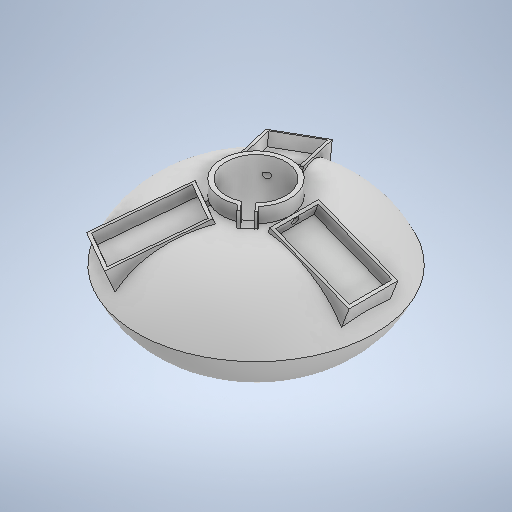
# Autodesk Inventor part: Water Sensor Bouy
Saved by Autodesk Inventor 2025 (Build 290162000, 162)
## iProperties
Created: 2024-06-17
Part Number: Water Sensor Bouy
Material: Generic
Document SubType Name: Modeling
Designer: track
Density: 1 g/cm^3
Appearance: Default
Author: track
## iProperties of the stored document Water Sensor Bouy_3DPrint.ipt
Created: 2024-06-17
Part Number: Water Sensor Bouy_3DPrint
Material: Generic
Document SubType Name: Modeling
Designer: track
Density: 1 g/cm^3
Appearance: Default
Author: track
Autodesk Inventor part; units mm, degrees
ref_plane "YZ Plane" through (0, 0, 0) normal (1, 0, 0) x (0, 1, 0)
ref_plane "XZ Plane" through (0, 0, 0) normal (0, 1, 0) x (-1, 0, 0)
ref_plane "XY Plane" through (0, 0, 0) normal (0, 0, 1) x (1, 0, 0)
sketch "Sketch1" plane through (0, 0, 0) normal (0, 0, 1) x (1, 0, 0)
  line L0 (0, 0) -> (0, 76.2)
  line L1 (25.3, 0) -> (25.3, 101.6)
  line L2 (25.3, 50.8) -> (101.5, 50.8)
  arc A0 (101.5, 50.8) -> (25.3, 101.6) centre (25.3, 19.05) ccw
  arc A1 (25.3, 0) -> (101.5, 50.8) centre (25.3, 82.55) ccw
  line L3 (35.3, 90.9075) -> (35.3, 10.6925)
  arc A2 (35.3, 10.6925) -> (90.5337, 50.8) centre (25.3, 82.55) ccw
  arc A3 (90.5337, 50.8) -> (35.3, 90.9075) centre (25.3, 19.05) ccw
  point P0 (25.3, 25.4)
  point P1 (84.8683, 25.4)
  point P2 (35.3, 31.75)
  point P3 (77.0964, 31.75)
  point P4 (35.3, 50.8)
  point P5 (90.5337, 50.8)
  point P6 (90.5337, 50.8)
  dimension "d0" = 101.6
  dimension "d1" = 25.3
  dimension "d2" = 50.8
  dimension "d3" = 0
  dimension "d4" = 76.2
  dimension "d24" = 82.55
  dimension "d33" = 10
  constraints: 10 point on circle, 8 end point, 4 centre point, 4 point on line, 2 vertical, 1 horizontal, 1 midpoint, 2 other
  measures "d0" distance of L1.start L1.end
  measures "d1" distance between parallel lines of L1 L0
  measures "d2" distance from line of L1.end L2
  measures "d3" vertical distance of L0.start L1.start
  measures "d4" distance of L2.start L2.end
  measures "d24" radius of A0
  measures "d33" distance between parallel lines of L1 L3
revolve "Revolution1" add sketch "Sketch1" angle 360 about axis through (0, 0, 0) along (0, 1, 0) contours L1 L2 L3 A2 A1 | L1 A0 L2 A3 L3
sketch "Sketch6" plane through (0, 0, 0) normal (0, 0, 1) x (1, 0, 0)
  arc A0 (101.5, 50.8) -> (25.3, 101.6) centre (25.3, 19.05) ccw projected
  line L0 (25.3, 101.6) -> (-25.3, 101.6) projected
  arc A1 (96.42, 60.96) -> (25.3, 101.6) centre (25.3, 19.05) ccw
  line L1 (55.0851, 96.0393) -> (28.9662, 50.8)
  line L2 (90.5337, 50.8) -> (-90.5337, 50.8) projected
  point P0 (0, 0)
  dimension "d34" = 60
  dimension "d35" = 12.7
  constraints: 4 point on circle, 2 end point, 1 centre point, 1 concentric, 1 point on line
  measures "d34" angle of L2 L1
  measures "d35" distance from line of A0.centre L1
ref_plane "Work Plane4" through (55.0851, 96.0393, 0) normal (0.3608127, 0.9326383, 0) x (-0.9326383, 0.3608127, 0)
sketch "Sketch17" plane through (55.0851, 96.0393, 0) normal (0.3608127, 0.9326383, 0) x (-0.9326383, 0.3608127, 0)
  line L0 (21.6308, 18.25) -> (-45.8692, 18.25)
  line L1 (-45.8692, 18.25) -> (-45.8692, -18.25)
  line L2 (-45.8692, -18.25) -> (21.6308, -18.25)
  line L3 (21.6308, -18.25) -> (21.6308, 18.25)
  ellipse E0 centre (53.3808, 0) end of major axis (53.3808, -25.3) minor radius 23.5957 projected
  point P0 (16.7223, 0)
  point P1 (21.6308, 0)
  dimension "d93" = 36.5
  dimension "d94" = 67.5
  dimension "d95" = 0
  dimension "d96" = 31.75
  constraints: 8 end point, 2 parallel, 1 horizontal, 1 midpoint, 1 perpendicular
  measures "d93" distance of L2.end L0.start
  measures "d94" distance of L1.end L2.end
  measures "d95" vertical distance of E0.centre point (21.631, 0)
  measures "d96" distance from line of E0.centre L3
extrude "Extrusion10" cut sketch "Sketch17" against normal blind 10 contours L3 L2 L1 L0
sketch "Sketch18" plane through (55.0851, 96.0393, 0) normal (0.3608127, 0.9326383, 0) x (-0.9326383, 0.3608127, 0)
  line L0 (21.6308, -18.25) -> (-36.2714, -18.25) projected
  line L1 (21.6308, -18.25) -> (-45.8692, -18.25)
  line L2 (-45.8692, -18.25) -> (-45.8692, 18.25)
  line L3 (-45.8692, 18.25) -> (21.6308, 18.25)
  line L4 (21.6308, 18.25) -> (21.6308, -18.25)
  line L5 (24.1708, -20.79) -> (-48.4092, -20.79)
  line L6 (-48.4092, -20.79) -> (-48.4092, 20.79)
  line L7 (-48.4092, 20.79) -> (24.1708, 20.79)
  line L8 (24.1708, 20.79) -> (24.1708, -20.79)
  point P0 (16.7223, 0)
  dimension "d99" = 36.5
  dimension "d100" = 67.5
  dimension "d101" = 2.54
  constraints: 16 end point, 4 parallel, 2 perpendicular, 1 horizontal, 3 other
  measures "d99" distance of L3.end L0.start
  measures "d100" distance of L0.start L1.end
  measures "d101" distance between parallel lines of L3 L7
extrude "Extrusion11" add sketch "Sketch18" against normal up to surface
sketch "Sketch19" plane through (51.477, 86.7129, 0) normal (0.3608127, 0.9326383, 0) x (0.9326383, -0.3608127, 0)
  line L0 (45.8692, -18.25) -> (-21.6308, -18.25) projected
  line L1 (-21.6308, 18.25) -> (36.2714, 18.25) projected
  line L2 (45.8692, -18.25) -> (-21.6308, -18.25)
  line L3 (-21.6308, -18.25) -> (-21.6308, 18.25)
  line L4 (-21.6308, 18.25) -> (45.8692, 18.25)
  line L5 (45.8692, 18.25) -> (45.8692, -18.25)
  point P0 (-16.7223, 0)
  point P1 (-21.6308, -18.25)
  constraints: 8 end point, 2 parallel, 1 horizontal, 1 perpendicular
extrude "Extrusion12" add sketch "Sketch19" against normal blind 10
sketch "Sketch20" plane through (0, 0, 0) normal (1, 0, 0) x (0, 1, 0)
  circle A0 centre (100.034, 0) radius 3
  line L0 (101.6, -25.3) -> (101.6, 25.3) projected
  line L1 (103.844, 18.25) -> (103.844, -18.25) projected
  line L2 (103.844, -18.25) -> (94.5176, -18.25) projected
  point P0 (0, 0)
  dimension "d106" = 6
  dimension "d108" = 3.81
  dimension "d109" = 18.25
  constraints: 1 centre point
  measures "d106" diameter of A0
  measures "d108" distance from line of L1 A0.centre
  measures "d109" distance from line of L2 A0.centre
extrude "Extrusion13" cut sketch "Sketch20" against normal up to surface surface through (34.9113, 103.844, 18.25) normal (-0.9326383, 0.3608127, 0)
pattern_circular "Circular Pattern4" count 3 over 360 about axis through (0, 50.8, 0) along (0, 1, 0) of "Extrusion13", "Extrusion12", "Extrusion11", "Extrusion10"
sketch "Sketch21" plane through (0, 0, 0) normal (1, 0, 0) x (0, 1, 0)
  arc A0 (50.8, -101.5) -> (101.6, -25.3) centre (19.05, -25.3) ccw projected
  arc A1 (50.8, -101.5) -> (101.6, -25.3) centre (19.05, -25.3) ccw
  line L0 (101.6, -25.3) -> (114.3, -25.3)
  line L1 (114.3, -25.3) -> (114.3, -29.11)
  line L2 (114.3, -29.11) -> (101.512, -29.11)
  line L3 (0, 0) -> (101.6, 0)
  line L4 (101.6, -20.5187) -> (101.6, 20.5187) projected
  dimension "d115" = 3.81
  dimension "d116" = 12.7
  dimension "d117" = 25.3
  dimension "d118" = 25.3
  constraints: 8 end point, 5 point on circle, 2 perpendicular, 1 centre point, 1 horizontal, 1 midpoint
  measures "d115" distance of L0.end L1.end
  measures "d116" distance of L0.start L0.end
  measures "d117" distance between parallel lines of L3 L0
  measures "d118" distance from line of L3 A0.centre
revolve "Revolution3" add sketch "Sketch21" angle 210 about axis through (0, 0, 0) along (0, 1, 0) and the other way 140
sketch "Sketch22" plane through (18.7115, 114.3, 22.2996) normal (0, 1, 0) x (0.7660444, 0, -0.6427876)
  line L0 (0, 29.11) -> (-2.205, 3.9063)
  arc A0 (0, 3.81) -> (-4.3933, 4.1944) centre (0, 29.11) ccw projected
  line L1 (0, 29.11) -> (0, 54.41)
  circle A1 centre (0, 29.11) radius 25.3
  dimension "d121" = 175
  constraints: 4 end point, 1 coincident, 1 point on circle, 1 vertical, 3 other
  measures "d121" angle of L1 L0
ref_plane "Work Plane5" through (14.5115, 114.3, 20.7245) normal (-0.7660444, 0, 0.6427876) x (0.6427876, 0, 0.7660444)
sketch "Sketch23" plane through (14.5115, 114.3, 20.7245) normal (-0.7660444, 0, 0.6427876) x (0.6427876, 0, 0.7660444)
  line L0 (-0.2881, -12.7) -> (-0.2881, 0) projected
  line L1 (-0.2881, 0) -> (8.6019, 0)
  line L2 (8.6019, 0) -> (8.6019, -15.24)
  line L3 (8.6019, -15.24) -> (-0.2881, -15.24)
  line L4 (-0.2881, -15.24) -> (-0.2881, 0)
  point P0 (-25.2037, -114.3)
  point P1 (-0.2881, -12.7)
  dimension "d122" = 8.89
  dimension "d123" = 15.24
  constraints: 8 end point, 2 parallel, 1 horizontal, 1 perpendicular
  measures "d122" distance of L0.end L1.end
  measures "d123" distance of L1.end L2.end
extrude "Extrusion14" add sketch "Sketch23" along normal mid plane 12.7
sketch "Sketch24" plane through (15.1763, 101.0432, 31.3957) normal (0.6427876, 0, 0.7660444) x (0.7660444, 0, -0.6427876)
  line L0 (33.855, 13.2568) -> (-16.745, 13.2568) projected
  line L1 (1.905, 13.2568) -> (10.795, 13.2568)
  line L2 (10.795, 13.2568) -> (10.795, -0.2814)
  line L3 (10.795, -0.2814) -> (1.905, -0.2814)
  line L4 (1.905, -0.2814) -> (1.905, 13.2568)
  line L5 (12.7, 13.2568) -> (12.7, 0.0908) projected
  line L6 (0, 0) -> (0, 13.2568) projected
  point P0 (8.555, -101.0432)
  point P1 (4.1617, 13.2568)
  point P2 (10.795, 13.2568)
  dimension "d126" = 1.905
  dimension "d127" = 1.905
  dimension "d128" = 13.5382
  constraints: 8 end point, 2 parallel, 1 horizontal, 1 perpendicular, 1 point on line
  measures "d126" distance between parallel lines of L5 L2
  measures "d127" distance between parallel lines of L6 L4
  measures "d128" distance of L1.end L2.end
extrude "Extrusion15" cut sketch "Sketch24" against normal blind 12.7
sketch "Sketch25" plane through (19.3759, 114.3, 16.6428) normal (0.7660444, 0, -0.6427876) x (-0.6427876, 0, -0.7660444)
  circle A0 centre (-6.0619, -2.54) radius 0.75
  circle A1 centre (-6.0619, -5.08) radius 0.75
  circle A2 centre (-6.0619, -7.62) radius 0.75
  line L0 (-8.6019, 0) -> (-8.6019, -13.166) projected
  line L1 (-3.6097, 0) -> (-8.6019, 0) projected
  point P0 (25.2037, -114.3)
  dimension "d131" = 2.54
  dimension "d132" = 2.54
  dimension "d133" = 1.5
  dimension "d134" = 1.5
  dimension "d135" = 1.5
  dimension "d136" = 2.54
  dimension "d137" = 2.54
  dimension "d138" = 2.54
  dimension "d139" = 2.54
  constraints: 3 centre point
  measures "d131" distance of A1.centre A0.centre
  measures "d132" distance of A1.centre A2.centre
  measures "d133" diameter of A0
  measures "d134" diameter of A1
  measures "d135" diameter of A2
  measures "d136" distance from line of L0 A0.centre
  measures "d137" distance from line of L0 A1.centre
  measures "d138" distance from line of L1 A0.centre
  measures "d139" distance from line of L0 A2.centre
extrude "Extrusion16" cut sketch "Sketch25" against normal up to surface (12.7 mm away)
sketch "Sketch26" plane through (0, 0, 0) normal (0, 1, 0) x (-1, 0, 0)
  line L0 (0, 0) -> (-13.716, 0)
  circle A0 centre (-63.5, 0) radius 3.175
  dimension "d142" = 6.35
  dimension "d143" = 63.5
  constraints: 2 end point, 1 centre point, 1 horizontal, 1 point on line
  measures "d142" diameter of A0
  measures "d143" distance of L0.start A0.centre
extrude "Extrusion17" cut sketch "Sketch26" along normal blind 25
pattern_circular "Circular Pattern5" count 3 over 360 about axis through (0, 82.55, 0) along (0, 1, 0) of "Extrusion17"
body "Solid1"
